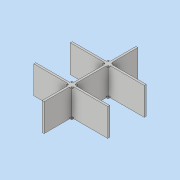
# Autodesk Inventor part: крепление-стенки
Saved by Autodesk Inventor 2019 (Build 230136000, 136)
## iProperties
Created: 2019-10-05
Part Number: крепление-стенки
Material: Типовые
Document SubType Name: Modeling
Designer: Iliga
Density: 1 g/cm^3
Appearance: По умолчанию
Author: Iliga
Autodesk Inventor part; units mm, degrees
ref_plane "YZ Plane" through (0, 0, 0) normal (1, 0, 0) x (0, 1, 0)
ref_plane "XY Plane" through (0, 0, 0) normal (0, 0, 1) x (1, 0, 0)
sketch "Эскиз1" plane through (0, 0, 0) normal (0, 1, 0) x (-1, 0, 0)
  line L0 (-2, 95) -> (2, 95)
  line L1 (2, 95) -> (2, -95)
  line L2 (2, -95) -> (-2, -95)
  line L3 (-2, -95) -> (-2, 95)
  line L4 (75, 35) -> (-75, 35)
  line L5 (-75, 35) -> (-75, 39)
  line L6 (-75, 39) -> (75, 39)
  line L7 (75, 39) -> (75, 35)
  line L8 (75, -35) -> (-75, -35)
  line L9 (-75, -35) -> (-75, -39)
  line L10 (-75, -39) -> (75, -39)
  line L11 (75, -39) -> (75, -35)
  line L12 (75, 35) -> (75, -35) construction
  line L13 (2, -95) -> (2, -95)
  line L14 (2, -95) -> (-2, -95)
  point P0 (0, 0)
  point P1 (0, -35)
  point P2 (75, 0)
  point P3 (0, -95)
  point P4 (2, 0)
  dimension "d1" = 150
  dimension "d3" = 4
  dimension "d4" = 4
  dimension "d5" = 4
  dimension "d26" = 35
  dimension "d27" = 35
  dimension "d28" = 95
  dimension "d29" = 95
  dimension "d32" = 56
  constraints: 30 end point, 5 parallel, 5 perpendicular, 4 midpoint, 3 horizontal, 3 point on line, 2 vertical alignment, 1 horizontal alignment
  measures "d1" distance between parallel lines of L5 L7
  measures "d3" distance between parallel lines of L6 L4
  measures "d4" distance between parallel lines of L1 L3
  measures "d5" distance between parallel lines of L10 L8
  measures "d26" distance from line of point (0, 0) L8
  measures "d27" distance from line of point (0, 0) L4
  measures "d28" distance from line of L0 point (0, 0)
  measures "d29" distance of point (0, -95) point (0, 0)
  measures "d32" distance from line of L0.start L6
extrude "Выдавливание1" add sketch "Эскиз1" along normal blind 56
ref_plane "РабПлоскость1" through (0, 28, 0) normal (0, 1, 0) x (-1, 0, 0)
sketch "Эскиз2" plane through (0, 0, 0) normal (0, 1, 0) x (-1, 0, 0)
  line L0 (-2, 39) -> (-2, 95) construction
  line L1 (-2, 95) -> (2, 95) construction
  line L2 (2, 95) -> (2, 39) construction
  line L3 (2, 39) -> (75, 39) construction
  line L4 (75, 39) -> (75, 35) construction
  line L5 (75, 35) -> (2, 35) construction
  line L6 (2, 35) -> (2, -35) construction
  line L7 (75, -35) -> (2, -35) construction
  line L8 (75, -39) -> (75, -35) construction
  line L9 (2, -39) -> (75, -39) construction
  line L10 (2, -39) -> (2, -95) construction
  line L11 (2, -95) -> (-2, -95) construction
  line L12 (-2, -95) -> (-2, -39) construction
  line L13 (-75, -39) -> (-2, -39) construction
  line L14 (-75, -35) -> (-75, -39) construction
  line L15 (-2, -35) -> (-75, -35) construction
  line L16 (-2, -35) -> (-2, 35) construction
  line L17 (-2, 35) -> (-75, 35) construction
  line L18 (-75, 35) -> (-75, 39) construction
  line L19 (-75, 39) -> (-2, 39) construction
  line L20 (-2, 35) -> (-6, 35)
  line L21 (-6, 35) -> (-6, 32)
  line L22 (-5, 31) -> (-2, 31)
  line L23 (-2, 31) -> (-2, 35)
  circle A0 centre (-4, 33) radius 1
  arc A1 (-6, 32) -> (-5, 31) centre (-5, 32) ccw
  line L24 (-2, -39) -> (-6, -39)
  line L25 (-6, -39) -> (-6, -42)
  line L26 (-5, -43) -> (-2, -43)
  line L27 (-2, -43) -> (-2, -39)
  circle A2 centre (-4, -41) radius 1
  arc A3 (-6, -42) -> (-5, -43) centre (-5, -42) ccw
  line L28 (-75, 37) -> (75, 37) construction
  line L29 (-75, -37) -> (75, -37) construction
  line L30 (0, 95) -> (0, -95) construction
  line L31 (-2, 39) -> (-6, 39)
  line L32 (-6, 39) -> (-6, 42)
  line L33 (-5, 43) -> (-2, 43)
  line L34 (-2, 43) -> (-2, 39)
  circle A4 centre (-4, 41) radius 1
  arc A5 (-5, 43) -> (-6, 42) centre (-5, 42) ccw
  line L35 (2, 35) -> (6, 35)
  line L36 (6, 35) -> (6, 32)
  line L37 (5, 31) -> (2, 31)
  line L38 (2, 31) -> (2, 35)
  circle A6 centre (4, 33) radius 1
  arc A7 (5, 31) -> (6, 32) centre (5, 32) ccw
  arc A8 (6, 42) -> (5, 43) centre (5, 42) ccw
  line L39 (5, 43) -> (2, 43)
  line L40 (2, 43) -> (2, 39)
  line L41 (6, 39) -> (6, 42)
  line L42 (2, 39) -> (6, 39)
  circle A9 centre (4, 41) radius 1
  line L43 (-2, -31) -> (-2, -35)
  line L44 (-2, -35) -> (-6, -35)
  circle A10 centre (-4, -33) radius 1
  line L45 (-6, -35) -> (-6, -32)
  arc A11 (-5, -31) -> (-6, -32) centre (-5, -32) ccw
  line L46 (-5, -31) -> (-2, -31)
  line L47 (2, -43) -> (2, -39)
  line L48 (2, -39) -> (6, -39)
  circle A12 centre (4, -41) radius 1
  line L49 (6, -39) -> (6, -42)
  arc A13 (5, -43) -> (6, -42) centre (5, -42) ccw
  line L50 (5, -43) -> (2, -43)
  line L51 (2, -31) -> (2, -35)
  line L52 (2, -35) -> (6, -35)
  line L53 (6, -35) -> (6, -32)
  line L54 (5, -31) -> (2, -31)
  arc A14 (6, -32) -> (5, -31) centre (5, -32) ccw
  circle A15 centre (4, -33) radius 1
  point P0 (0, 0)
  point P1 (-6, 31)
  point P2 (-6, -43)
  point P3 (-6, 43)
  point P4 (6, 31)
  point P5 (6, 43)
  point P6 (-6, -31)
  point P7 (2, -35)
  point P8 (6, -43)
  point P9 (6, -31)
  dimension "d11" = 4
  dimension "d12" = 4
  dimension "d13" = 2
  dimension "d15" = 1
  dimension "d16" = 2
  dimension "d17" = 2
  dimension "d18" = 4
  dimension "d19" = 4
  dimension "d20" = 2
  dimension "d21" = 1
  dimension "d22" = 2
  dimension "d23" = 2
  constraints: 70 end point, 49 symmetric about line, 18 point on line, 16 centre point, 16 point on circle, 6 midpoint, 4 parallel, 4 tangent, 2 horizontal, 2 perpendicular, 12 other
  measures "d11" distance of L22.end point (-6, 31)
  measures "d12" distance of point (-6, 31) L20.end
  measures "d13" diameter of A0
  measures "d15" radius of A1
  measures "d16" distance from line of L20 A0.centre
  measures "d17" distance from line of L23 A0.centre
  measures "d18" distance of L27.start point (-6, -43)
  measures "d19" distance of point (-6, -43) L24.end
  measures "d20" diameter of A2
  measures "d21" radius of A3
  measures "d22" distance from line of L24 A2.centre
  measures "d23" distance from line of L27 A2.centre
extrude "Выдавливание2" add sketch "Эскиз2" along normal blind 2
mirror "Зеркальное отражение1" about plane through (0, 28, 0) normal (0, 1, 0) of "Выдавливание2"
extrude "Выдавливание3" add sketch "Эскиз1" along normal up to surface (56 mm away) contours L0 L1 L6 L3 | L6 L1 L4 L3 | L4 L1 L8 L3 | L8 L1 L10 L3 | L10 L1 L2 L3
